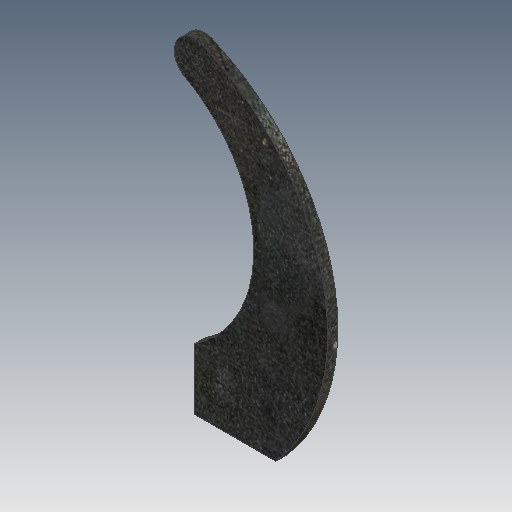
# Autodesk Inventor part: Halterung hinten unten
Saved by Autodesk Inventor 2020 (Build 240168000, 168)
## iProperties
Created: 2021-06-30
Part Number: Halterung hinten unten
Material: Stahl
Document SubType Name: Modeling
Designer: mike8
Density: 7.85 g/cm^3
Appearance: Platte
Mass: 244.009 g
Surface Area: 146.523 cm^2
Volume: 31.0839 cm^3
Author: mike8
Autodesk Inventor part; units mm, degrees
ref_plane "YZ Plane" through (0, 0, 0) normal (1, 0, 0) x (0, 1, 0)
ref_plane "XZ Plane" through (0, 0, 0) normal (0, 1, 0) x (-1, 0, 0)
ref_plane "XY Plane" through (0, 0, 0) normal (0, 0, 1) x (1, 0, 0)
sketch "Skizze1" plane through (0, 0, 0) normal (0, 0, 1) x (1, 0, 0)
  line L0 (-113.5762, 0) -> (48.979, 0) projected
  line L1 (0, -73.4285) -> (0, 160.1129) projected
  line L2 (-54.5088, -40.0654) -> (-14.5088, -40.0654)
  line L3 (-54.5088, -40.0654) -> (-54.5088, -10.0654)
  circle A0 centre (-54.5088, 109.9346) radius 10
  arc A1 (-14.5088, -40.0654) -> (-48.6674, 118.0511) centre (-89.0676, 26.5753) ccw
  arc A2 (-54.5088, -10.0654) -> (-60.3511, 101.8187) centre (-90.354, 44.1574) ccw
  point P0 (0, 0)
  point P1 (-58.162, 100.6258)
  dimension "d0" = 30
  dimension "d1" = 40
  dimension "d6" = 150
  dimension "d7" = 20
  dimension "d8" = 65
  dimension "d9" = 100
  dimension "d10" = 0
  constraints: 6 point on circle, 4 end point, 3 centre point, 1 horizontal, 1 vertical
  measures "d0" distance of L2.start L3.end
  measures "d1" distance of L2.start L2.end
  measures "d6" distance from line of A0.centre L2
  measures "d7" diameter of A0
  measures "d8" radius of A2
  measures "d9" radius of A1
  measures "d10" distance from line of L3 A0.centre
extrude "Extrusion1" add sketch "Skizze1" along normal blind 5 contours A2 A0 A1 L1 L0 | L0 L1 A1 L2 L3 A2 | L1 A1 L0 | L0 A1 L1 | A2 A0 picked at (-52.7779, 112.7657)
sketch "Skizze2" plane through (0, 0, 5) normal (0, 0, 1) x (1, 0, 0)
  arc A0 (-48.6674, 118.0511) -> (-60.3511, 101.8187) centre (-54.5088, 109.9346) ccw projected
  point P0 (0, 0)
  dimension "d13" = 0
  dimension "d14" = 0
  measures "d13" distance of A0.centre point (-54.509, 109.935)
  measures "d14" distance of A0.centre point (-54.509, 109.935)
hole "Bohrung1" at (-54.5088, 109.9346, 5) direction (0, 0, -1) diameter 3 end through all
sketch "Skizze3" plane through (0, 0, 5) normal (0, 0, 1) x (1, 0, 0)
  line L0 (-54.5088, -40.0654) -> (-14.5088, -40.0654) projected
  arc A0 (-54.5088, -10.0654) -> (-60.3511, 101.8187) centre (-90.354, 44.1574) ccw projected
  point P0 (0, 0)
  point P1 (-5.354, 49.9346)
  dimension "d22" = 90
  dimension "d23" = 85
  measures "d22" distance from line of L0 point (-5.354, 49.935)
  measures "d23" horizontal distance of A0.centre point (-5.354, 49.935)
hole "Bohrung2" at (-5.354, 49.9346, 5) direction (0, 0, -1) diameter 3 end through all
